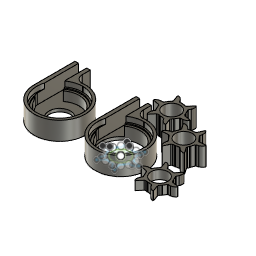
2020_09_27_3018 Motor to air blower v7 (Autodesk Fusion 360 design; units mm, degrees)
Autodesk Fusion 360 part; units mm, degrees
sketch "BlowerHolder" plane through (0, 0, 0) normal (0, 0, 1) x (1, 0, 0)
  circle A0 centre (0, 0) radius 21
  circle A1 centre (0, 0) radius 22.5
  line L0 (0, 0) -> (-22.5, 0) construction
  line L1 (-22.5, 0) -> (-22.5, 40)
  line L2 (-22.5, 40) -> (-12.5, 40)
  line L3 (-12.5, 40) -> (-12.5, 32.1932)
  line L4 (0, 0) -> (0, 1.7479)
  line L5 (0, 1.7479) -> (0, 22.5) construction
  line L6 (-12.5, 40) -> (0, 22.5) construction
  line L7 (0.4356, 22.6338) -> (0, 22.5)
  arc A2 (-12.5, 32.1932) -> (0.4356, 22.6338) centre (-2.5, 32.1932) ccw
  line L8 (-21.5, 0) -> (-21.5, 39)
  line L9 (-21.5, 39) -> (-13.5, 39)
  line L10 (-13.5, 39) -> (-13.5, 32.1932)
  arc A3 (-13.5, 32.1932) -> (0.7291, 21.6778) centre (-2.5, 32.1932) ccw
  arc A4 (0.7291, 21.6778) -> (0.142, 23.5897) centre (0.4356, 22.6338) ccw
  line L11 (0.142, 23.5897) -> (-0.2936, 23.4559)
  circle A5 centre (0, 0) radius 19
  line L12 (-13.5, 32.1932) -> (-13.5, 20.5093)
  line L13 (-12.0669, 15.9402) -> (-11.4996, 15.1248)
  arc A6 (-13.5, 20.5093) -> (-12.0669, 15.9402) centre (-5.5, 20.5093) ccw
  circle A7 centre (0, 0) radius 25
  line L14 (-21.5, 0) -> (-21.5, -0.5919)
  line L15 (-20.642, -3.3927) -> (-15.7394, -10.6429)
  arc A8 (-21.5, -0.5919) -> (-20.642, -3.3927) centre (-16.5, -0.5919) ccw
  line L16 (-25, 0) -> (-25, 40)
  line L17 (-10, 40) -> (-10, 32.1932)
  arc A9 (-10, 32.1932) -> (-0.2983, 25.0236) centre (-2.5, 32.1932) ccw
  arc A10 (1.1695, 20.2439) -> (-0.2983, 25.0236) centre (0.4356, 22.6338) ccw
  line L18 (1.1695, 20.2439) -> (0.7339, 20.1101)
  line L19 (-22.5, 40) -> (-25, 40)
  line L20 (-12.5, 40) -> (-10, 40)
  line L21 (-21.5, 39) -> (-21.5, 40)
  line L22 (-13.5, 39) -> (-13.5, 40)
  dimension "d1" = 42
  dimension "d2" = 45
  dimension "d3" = 40
  dimension "d4" = 10
  dimension "d5" = 10
  dimension "d6" = 1
  dimension "d7" = 38
  dimension "d8" = 8
  dimension "d14" = 50
  dimension "d17" = 5
  constraint coincident A0.centre A1.centre
  constraint coincident A1 L0.end
  constraint horizontal L0
  constraint perpendicular L0 L1
  constraint perpendicular L1 L2
  constraint perpendicular L2 L3
  constraint perpendicular L0 L4
  constraint coincident A1 L5.end
  constraint perpendicular L0 L5
  constraint tangent L7 A2
  constraint tangent L3 A2
  constraint concentric A1 A5
  constraint tangent A3 L12
  constraint vertical L12
  constraint coincident A5 L13.end
  constraint tangent L13 A6
  constraint tangent L12 A6
  constraint concentric A5 A7
  constraint coincident A5 L15.end
  constraint tangent A5 L15
  constraint tangent L15 A8
  constraint tangent L14 A8
  constraint perpendicular L16 L19
  constraint perpendicular L17 L20
  constraint parallel L1 L16
  constraint parallel L3 L17
  constraint concentric A2 A9
  constraint coincident L7.start A2.end
  constraint parallel L7 L18
  constraint tangent A9 A10
  constraint tangent A10 L18
  constraint tangent L17 A9
  constraint coincident L2 L21.end
  constraint perpendicular L2 L21
  constraint coincident L2 L22.end
  constraint perpendicular L2 L22
  measures "d1" diameter of A0
  measures "d2" diameter of A1
  measures "d3" distance of L0.end L1.end
  measures "d4" distance of L1.end L2.end
  measures "d5" radius of A2
  measures "d7" diameter of A5
  measures "d8" radius of A6
  measures "d14" diameter of A7
  measures "d17" radius of A8
extrude "Extrude1" add sketch "BlowerHolder" along normal blind 13 contours A0 A1 L8 L14 A8 A10 | A0 A1 A3 A4 A6 A10 | A0 A1 L8 A6 L14 A8 | A1 L1 A7 A10 | A1 L7 A2 A7 A9 A10 | A1 A3 L12 A6 A7 | A1 L8 L12 A6 A7 | A1 A2 A3 A4 | A1 A2 A3 A7 | A1 L1 L8 A7 | A1 A2 | A3 L12 A7 | L2 L3 A2 L10 A3 A7 L22 | L1 L2 L8 A7 L21 | L8 L9 L10 L12 A7 | L1 A7 L16 L19 | L3 A2 A7 L17 A9 L20 | L2 L9 L21 L22 makes body 1
extrude "Extrude2" add sketch "BlowerHolder" along normal blind 12 contours A0 A5 L13 A6 L15 A8 | A0 A5 L13 A6 L15 A8 bodies 1
extrude "Extrude3" add sketch "BlowerHolder" along normal blind 18 separate body contours A1 L1 A7 A10 | A1 L7 A2 A7 A9 A10 | A1 A3 L12 A6 A7 | A1 A2 A3 A7 | A1 L1 L8 A7 | A7 A9 | A3 L12 A7 | L2 L3 A2 L10 A3 A7 L22 | L1 L2 L8 A7 L21 | L1 A7 L16 L19 | L3 A2 A7 L17 A9 L20 makes body 2
extrude "Extrude4" cut sketch "BlowerHolder" along normal blind 18 contours A0 A1 L8 A6 L14 A8 | A0 A5 L13 A6 L15 A8 | A1 L8 L12 A6 A7 | L8 L9 L10 L12 A7 | L2 L9 L21 L22 picked at (-20.2431, -1.4827) bodies 1
sketch "Holes" plane through (0, 0, 0) normal (0, 0, 1) x (1, 0, 0)
  circle A0 centre (0, 0) radius 17.5
  circle A1 centre (0, 0) radius 10.5
  ellipse E0 centre (-10.4997, -0.0834) end of major axis (-17.499, -0.3278) minor radius 2.903 (-10.8794, 2.8058) -> (-17.4958, -0.3825) ccw
  line L0 (-17.4958, -0.3825) -> (-11.452, -1.4911)
  line L1 (0, 0) -> (-9.7843, -3.8103) construction
  line L2 (-9.7843, -3.8103) -> (-10.3248, -2.4222)
  arc A2 (-10.3248, -2.4222) -> (-11.452, -1.4911) centre (-11.7226, -2.9665) ccw
  line L3 (0, 0) -> (-8.7477, 5.8075) construction
  line L4 (-8.7477, 5.8075) -> (-10.5963, 3.0231)
  line L5 (-10.8794, 2.8058) -> (-10.9872, 2.8003)
  line L6 (-6.9278, 3.0092) -> (-6.6498, 2.5797) construction
  arc A3 (-10.9872, 2.8003) -> (-10.5963, 3.0231) centre (-11.0129, 3.2996) ccw
  circle A4 centre (0, 0) radius 8.25
  circle A5 centre (0, 0) radius 7.1
  dimension "d21" = 21
  dimension "d22" = 1.5
  dimension "d23" = 0.5115
  dimension "d24" = 0.5
  dimension "d35" = 16.5
  dimension "d36" = 35
  dimension "d37" = 14.2
  constraint coincident A0.centre A1.centre
  constraint coincident A1 E0.centre
  constraint coincident A0 L0.start
  constraint coincident A1 L1.end
  constraint tangent A1 L2
  constraint tangent L2 A2
  constraint tangent L0 A2
  constraint coincident A1 L3.end
  constraint tangent A1 L4
  constraint tangent E0 L5
  constraint coincident L6.start L5
  constraint tangent L5 A3
  constraint tangent L4 A3
  constraint concentric A1 A4
  constraint concentric A0 A5
  measures "d21" diameter of A1
  measures "d22" radius of A2
  measures "d23" distance of L6.start L6.end
  measures "d24" radius of A3
  measures "d35" diameter of A4
  measures "d36" diameter of A0
  measures "d37" diameter of A5
extrude "Extrude5" add sketch "Holes" along normal blind 8.5 separate body contours A0 A1 E0 L0 L2 A2 L4 L5 A3 picked at (-14.9299, -0.0782) makes body 3
pattern_circular "C-Pattern1" count 6 over 360 about axis through (0, 0, 1.75) along (0, 0, 1) of bodies 3 makes body 4 at (-9.1806, -5.0957, 2.8333) makes body 5 at (-0.1773, -10.4985, 2.8333) makes body 6 at (9.0033, -5.4028, 2.8333) makes body 7 at (9.1806, 5.0957, 2.8333) makes body 8 at (0.1773, 10.4985, 2.8333)
extrude "Extrude6" add sketch "Holes" along normal blind 8.5 separate body contours A1 | A4 | A5 makes body 9
combine "Combine1" operation add target body 9 tool bodies 3 8 6 5 4 7
extrude "Extrude7" cut sketch "Holes" along normal blind 18 contours A4 | A5 bodies 9
extrude "Extrude9" add sketch "BlowerHolder" along normal blind 3 contours A0 A1 L8 A6 L14 A8 | A0 A5 L13 A6 L15 A8 | A1 L8 L12 A6 A7 | A5 | L8 L9 L10 L12 A7 picked at (-20.2431, -1.4827) bodies 1 2
extrude "Extrude10" cut sketch "Holes" along normal blind 5 contours A1 | A4 | A5 bodies 1
extrude "Extrude12" add sketch "BlowerHolder" along normal blind 2 separate body contours A1 L1 A7 A10 | A1 L7 A2 A7 A9 A10 | A1 A3 L12 A6 A7 | A1 L8 L12 A6 A7 | A7 A9 A10 | A1 A2 A3 A7 | A1 L1 L8 A7 | A7 A9 | A3 L12 A7 | L2 L3 A2 L10 A3 A7 L22 | L1 L2 L8 A7 L21 | L8 L9 L10 L12 A7 | L1 A7 L16 L19 | L3 A2 A7 L17 A9 L20 | L2 L9 L21 L22 makes body 10
move_body "Move2" bodies 10 to x (1, 0, 0) y (0, 1, 0) z (0, 0, 1) at (0, 0, 18)
move_body "Move4" bodies 9 to x (1, 0, 0) y (0, 1, 0) z (0, 0, 1) at (0, 0, 3)
sketch "BladeSketch" plane through (0, 0, 0) normal (0, 0, 1) x (-1, 0, 0)
  circle A0 centre (0, 0) radius 8.25
  arc A1 (10.418, 2.4585) -> (11.47, 1.5895) centre (11.7226, 2.9665) ccw
  line L0 (17.5938, 0.4662) -> (11.47, 1.5895)
  arc A2 (17.5985, 0.2296) -> (17.5938, 0.4662) centre (0, 0) ccw
  spline S0 degree 3 poles (13.4152, -2.5752) (13.8769, -2.4732) (14.318, -2.3539) (14.7258, -2.2155) (16.4435, -1.6325) (17.5573, -0.7253) (17.5985, 0.2296) knots -1.159006 -1.159006 -1.159006 -1.159006 -0.942845 -0.942845 -0.942845 -0.032324 -0.032324 -0.032324 -0.032324
  line L1 (11.2306, -2.6876) -> (13.4152, -2.5752)
  line L2 (8.831, -5.8628) -> (10.7615, -2.955)
  arc A3 (8.2699, -6.6308) -> (8.831, -5.8628) centre (0, 0) ccw
  line L3 (7.3381, -7.793) -> (8.2699, -6.6308)
  arc A4 (7.3381, -7.793) -> (7.1115, -9.1386) centre (8.4304, -8.6688) ccw
  line L4 (9.2006, -15.0036) -> (7.1115, -9.1386)
  arc A5 (8.9981, -15.1259) -> (9.2006, -15.0036) centre (0, 0) ccw
  spline S1 degree 3 poles (4.4774, -12.9055) (4.7966, -13.2543) (5.1205, -13.5767) (5.4442, -13.8607) (6.808, -15.0567) (8.1505, -15.5677) (8.9981, -15.1259) knots -1.159006 -1.159006 -1.159006 -1.159006 -0.942845 -0.942845 -0.942845 -0.032324 -0.032324 -0.032324 -0.032324
  line L5 (3.2877, -11.0698) -> (4.4774, -12.9055)
  line L6 (-0.6619, -10.5793) -> (2.8217, -10.7973)
  arc A6 (-1.6075, -10.4774) -> (-0.6619, -10.5793) centre (0, 0) ccw
  line L7 (-3.0799, -10.2515) -> (-1.6075, -10.4774)
  arc A7 (-3.0799, -10.2515) -> (-4.3585, -10.728) centre (-3.2922, -11.6353) ccw
  line L8 (-8.3932, -15.4698) -> (-4.3585, -10.728)
  arc A8 (-8.6004, -15.3556) -> (-8.3932, -15.4698) centre (0, 0) ccw
  spline S2 degree 3 poles (-8.9378, -10.3303) (-9.0803, -10.7811) (-9.1975, -11.2228) (-9.2816, -11.6452) (-9.6355, -13.4243) (-9.4068, -14.8424) (-8.6004, -15.3556) knots -1.159006 -1.159006 -1.159006 -1.159006 -0.942845 -0.942845 -0.942845 -0.032324 -0.032324 -0.032324 -0.032324
  line L9 (-7.9428, -8.3822) -> (-8.9378, -10.3303)
  line L10 (-9.4929, -4.7165) -> (-7.9398, -7.8423)
  arc A9 (-9.8775, -3.8465) -> (-9.4929, -4.7165) centre (0, 0) ccw
  line L11 (-10.418, -2.4585) -> (-9.8775, -3.8465)
  arc A10 (-10.418, -2.4585) -> (-11.47, -1.5895) centre (-11.7226, -2.9665) ccw
  line L12 (-17.5938, -0.4662) -> (-11.47, -1.5895)
  arc A11 (-17.5985, -0.2296) -> (-17.5938, -0.4662) centre (0, 0) ccw
  spline S3 degree 3 poles (-13.4152, 2.5752) (-13.8769, 2.4732) (-14.318, 2.3539) (-14.7258, 2.2155) (-16.4435, 1.6325) (-17.5573, 0.7253) (-17.5985, -0.2296) knots -1.159006 -1.159006 -1.159006 -1.159006 -0.942845 -0.942845 -0.942845 -0.032324 -0.032324 -0.032324 -0.032324
  line L13 (-11.2306, 2.6876) -> (-13.4152, 2.5752)
  line L14 (-8.831, 5.8628) -> (-10.7615, 2.955)
  arc A12 (-8.2699, 6.6308) -> (-8.831, 5.8628) centre (0, 0) ccw
  line L15 (-7.3381, 7.793) -> (-8.2699, 6.6308)
  arc A13 (-7.3381, 7.793) -> (-7.1115, 9.1386) centre (-8.4304, 8.6688) ccw
  line L16 (-9.2006, 15.0036) -> (-7.1115, 9.1386)
  arc A14 (-8.9981, 15.1259) -> (-9.2006, 15.0036) centre (0, 0) ccw
  spline S4 degree 3 poles (-4.4774, 12.9055) (-4.7966, 13.2543) (-5.1205, 13.5767) (-5.4442, 13.8607) (-6.808, 15.0567) (-8.1505, 15.5677) (-8.9981, 15.1259) knots -1.159006 -1.159006 -1.159006 -1.159006 -0.942845 -0.942845 -0.942845 -0.032324 -0.032324 -0.032324 -0.032324
  line L17 (-3.2877, 11.0698) -> (-4.4774, 12.9055)
  line L18 (0.6619, 10.5793) -> (-2.8217, 10.7973)
  arc A15 (1.6075, 10.4774) -> (0.6619, 10.5793) centre (0, 0) ccw
  line L19 (3.0799, 10.2515) -> (1.6075, 10.4774)
  arc A16 (3.0799, 10.2515) -> (4.3585, 10.728) centre (3.2922, 11.6353) ccw
  line L20 (8.3932, 15.4698) -> (4.3585, 10.728)
  arc A17 (8.6004, 15.3556) -> (8.3932, 15.4698) centre (0, 0) ccw
  spline S5 degree 3 poles (8.9378, 10.3303) (9.0803, 10.7811) (9.1975, 11.2228) (9.2816, 11.6452) (9.6355, 13.4243) (9.4068, 14.8424) (8.6004, 15.3556) knots -1.159006 -1.159006 -1.159006 -1.159006 -0.942845 -0.942845 -0.942845 -0.032324 -0.032324 -0.032324 -0.032324
  line L21 (7.9428, 8.3822) -> (8.9378, 10.3303)
  line L22 (9.4929, 4.7165) -> (7.9398, 7.8423)
  arc A18 (9.8775, 3.8465) -> (9.4929, 4.7165) centre (0, 0) ccw
  line L23 (10.418, 2.4585) -> (9.8775, 3.8465)
  arc A19 (11.2306, -2.6876) -> (10.7615, -2.955) centre (11.2614, -3.2868) ccw
  arc A20 (3.2877, -11.0698) -> (2.8217, -10.7973) centre (2.7842, -11.3961) ccw
  arc A21 (-7.9428, -8.3822) -> (-7.9398, -7.8423) centre (-8.4772, -8.1093) ccw
  arc A22 (-11.2306, 2.6876) -> (-10.7615, 2.955) centre (-11.2614, 3.2868) ccw
  arc A23 (-3.2877, 11.0698) -> (-2.8217, 10.7973) centre (-2.7842, 11.3961) ccw
  arc A24 (7.9428, 8.3822) -> (7.9398, 7.8423) centre (8.4772, 8.1093) ccw
  dimension "d63" = 0.6
  constraint tangent A1 L23
  constraint tangent A1 L0
  constraint tangent L2 A3
  constraint tangent L3 A4
  constraint tangent A3 L3
  constraint tangent A4 L4
  constraint tangent A10 L12
  constraint tangent L22 A18
  constraint tangent L15 A13
  constraint tangent L6 A6
  constraint tangent A6 L7
  constraint tangent L7 A7
  constraint tangent A7 L8
  constraint tangent L10 A9
  constraint tangent A9 L11
  constraint tangent L11 A10
  constraint tangent L14 A12
  constraint tangent A12 L15
  constraint tangent A13 L16
  constraint tangent A18 L23
  constraint tangent L19 A16
  constraint tangent L18 A15
  constraint tangent A15 L19
  constraint tangent A16 L20
  constraint tangent L1 A19
  constraint tangent L2 A19
  constraint tangent L5 A20
  constraint tangent L6 A20
  constraint equal A19 A20
  constraint tangent L9 A21
  constraint tangent L10 A21
  constraint equal A19 A21
  constraint tangent L13 A22
  constraint tangent L14 A22
  constraint equal A19 A22
  constraint tangent L17 A23
  constraint tangent L18 A23
  constraint equal A19 A23
  constraint tangent L21 A24
  constraint tangent L22 A24
  constraint equal A19 A24
  measures "d63" radius of A19
extrude "Extrude16" add sketch "BladeSketch" along normal blind 8.5 separate body makes body 11
copy_body "CopyPasteBodies1" bodies 1 makes body 12
extrude "Extrude18" cut sketch "BlowerHolder" along normal blind 18 contours A5 bodies 12
extrude "Extrude19" add sketch "BladeSketch" along normal blind 18 separate body makes body 13
move_body "Move6" bodies 13 to x (1, 0, 0) y (0, 1, 0) z (0, 0, 1) at (55, 0, 0)
move_body "Move7" bodies 11 to x (1, 0, 0) y (0, 1, 0) z (0, 0, 1) at (55, 34, 0)
move_body "Move8" bodies 1 to x (1, 0, 0) y (0, 1, 0) z (0, 0, 1) at (-60, 0, 0)
move_body "Move9" bodies 13 to x (1, 0, 0) y (0, 1, 0) z (0, 0, 1) at (-50, 45, 0)
copy_body "CopyPasteBodies2" bodies 13 makes body 14
move_body "Move10" bodies 14 to x (1, 0, 0) y (0, 1, 0) z (0, 0, 1) at (30, -10, 0)
move_body "Move11" bodies 11 to x (1, 0, 0) y (0, 1, 0) z (0, 0, 1) at (-10, -30, 0)
move_body "Move12" bodies 13 to x (1, 0, 0) y (0, 1, 0) z (0, 0, 1) at (-1, 1, 0)
move_face "MoveFace2" by (0, -2, 0) 1 faces at (45.2204, 34.647, 18) on bodies 14
move_body "Move13" bodies 14 to x (0.34202, 0.939693, 0) y (-0.939693, 0.34202, 0) z (0, 0, 1) at (55.9185, -9.8599, 0)
move_body "Move14" bodies 14 to x (1, 0, 0) y (0, 1, 0) z (0, 0, 1) at (-5, -7, 0)
move_body "Move15" bodies 14 to x (0.996195, 0.087156, 0) y (-0.087156, 0.996195, 0) z (0, 0, 1) at (2.5545, -2.5081, 0)
move_body "Move16" bodies 11 to x (1, 0, 0) y (0, 1, 0) z (0, 0, 1) at (0, -11, 0)
move_body "Move17" bodies 14 to x (1, 0, 0) y (0, 1, 0) z (0, 0, 1) at (2, 1, 0)
move_body "Move18" bodies 14 to x (1, 0, 0) y (0, 1, 0) z (0, 0, 1) at (2, -1, 0)
hidden bodies 9 10
equation "WoodHeight = 18 mm"
equation "d10 = WoodHeight - 5 mm"
equation "d12 = WoodHeight - 6 mm"
equation "d15 = WoodHeight"
equation "d18 = WoodHeight"
equation "d25 = ThinBlade"
equation "d31 = ThinBlade"
equation "d41 = WoodHeight"
equation "ThinBlade = 8.5 mm"
equation "d61 = ThinBlade"
equation "d66 = WoodHeight"
equation "ThickBlade = 18 mm"
equation "d69 = ThickBlade"
named bodies: "Blower", "TopCover", "Blade", "Thin Blade", "Blower Compartement", "Thick Blade", "Thick Blade (1)"
